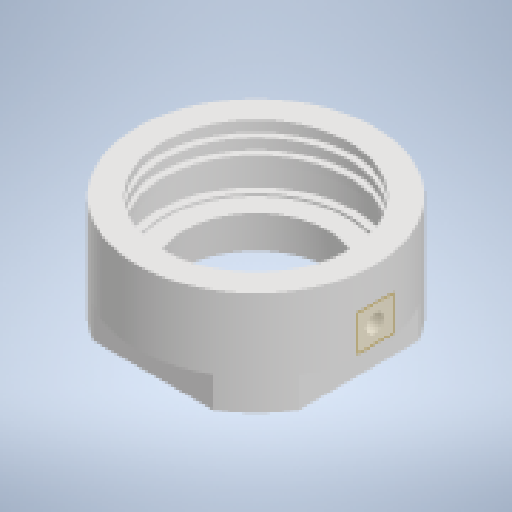
# Autodesk Inventor part: WashChamberConduit_1
Saved by Autodesk Inventor 2024 (Build 280153000, 153)
## iProperties
Created: 2025-02-06
Part Number: WashChamberConduit_1
Material: Generic
Document SubType Name: Modeling
Designer: Tommy Rohmann
Density: 1 g/cm^3
Appearance: Default
Author: Tommy Rohmann
Autodesk Inventor part; units mm, degrees
ref_plane "YZ Plane" through (0, 0, 0) normal (1, 0, 0) x (0, 1, 0)
ref_plane "XZ Plane" through (0, 0, 0) normal (0, 1, 0) x (-1, 0, 0)
ref_plane "XY Plane" through (0, 0, 0) normal (0, 0, 1) x (1, 0, 0)
sketch "WashChamberConduit" plane through (0, 0, 0) normal (0, 0, 1) x (1, 0, 0)
  line L0 (57.15, 1.0107) -> (61.9125, 1.0107)
  line L1 (57.15, -2.1643) -> (57.15, 31.7898)
  line L2 (57.785, 35.3007) -> (61.9125, 35.3007)
  line L3 (61.9125, 35.3007) -> (61.9125, 30.5382)
  line L4 (61.9125, 30.5382) -> (57.785, 30.5382)
  line L5 (57.785, 30.5382) -> (57.785, 25.7757)
  line L6 (57.785, 25.7757) -> (61.9125, 25.7757)
  line L7 (61.9125, 25.7757) -> (61.9125, 21.0132)
  line L8 (61.9125, 1.0107) -> (61.9125, 16.2507)
  line L9 (57.785, 35.3007) -> (57.785, 40.0632)
  line L10 (57.785, 40.0632) -> (73.9267, 40.0632)
  line L11 (73.9267, -5.3393) -> (63.7667, -5.3393)
  line L12 (63.7667, -5.3393) -> (63.7667, -24.3893)
  line L13 (61.9125, 21.0132) -> (57.785, 21.0132)
  line L14 (57.785, 21.0132) -> (57.785, 16.2507)
  line L15 (57.785, 16.2507) -> (61.9125, 16.2507)
  line L16 (0, 0) -> (0, 25.5104)
  line L17 (73.9267, -5.3393) -> (73.9267, 40.0632)
  line L18 (57.15, 1.0107) -> (57.15, -0.5768)
  line L19 (63.7667, -24.3893) -> (73.9267, -24.3893)
  line L20 (73.9267, -24.3893) -> (73.9267, -5.3393)
  line L21 (61.9125, 8.6307) -> (73.9267, 8.6307)
  line L22 (57.15, 1.0107) -> (63.8852, 1.0107)
  line L23 (57.15, -0.5768) -> (44.45, -0.5768)
  line L24 (44.45, -0.5768) -> (46.0375, -8.5143)
  line L25 (46.0375, -8.5143) -> (47.625, -16.4518)
  line L26 (47.625, -16.4518) -> (49.2125, -24.3893)
  line L27 (63.7667, -24.3893) -> (49.2125, -24.3893)
  point P0 (52.07, -10.4939)
  dimension "d9" = 0.635
  dimension "d12" = 4.7625
  dimension "d13" = 4.7625
  dimension "d17" = 15.24
  dimension "d41" = 10.16
  dimension "d42" = 12.0142
  dimension "d44" = 114.3
  dimension "WashConduitOD" = 147.8534
  dimension "d46" = 1.5875
  dimension "d65" = 19.05
  dimension "d232" = 92.075
  dimension "d233" = 95.25
  dimension "d234" = 23.8125
  dimension "ConduitHatchAngle" = 78.69
  dimension "ConduitHatchID" = 88.9
  measures "d9" distance between parallel lines of L1 L9
  measures "d12" distance between parallel lines of L1 L3
  measures "d13" distance between parallel lines of L2 L10
  measures "d17" distance between parallel lines of L15 L0
  measures "d41" distance between parallel lines of L17 L12
  measures "d42" distance between parallel lines of L17 L8
  measures "d44" diameter of L1 L16
  measures "WashConduitOD" diameter of L17 L16
  measures "d46" distance of L0.start L18.end
  measures "d65" distance between parallel lines of L19 L11
  measures "d232" diameter of L24.end L16
  measures "d233" diameter of L25.end L16
  measures "d234" distance from line of L23.end L27
  measures "ConduitHatchAngle" angle of L23 L24
  measures "ConduitHatchID" diameter of L23.end L16
derived "WashChamberLayout.ipt"
sketch "Sketch1" plane through (0, 0, 0) normal (0, 0, 1) x (1, 0, 0)
  line L0 (57.15, 1.0107) -> (61.9125, 1.0107)
  line L1 (57.15, -2.1643) -> (57.15, 31.7898)
  line L2 (57.785, 35.3007) -> (61.9125, 35.3007)
  line L3 (61.9125, 35.3007) -> (61.9125, 30.5382)
  line L4 (61.9125, 30.5382) -> (57.785, 30.5382)
  line L5 (57.785, 30.5382) -> (57.785, 25.7757)
  line L6 (57.785, 25.7757) -> (61.9125, 25.7757)
  line L7 (61.9125, 25.7757) -> (61.9125, 21.0132)
  line L8 (61.9125, 1.0107) -> (61.9125, 16.2507)
  line L9 (57.785, 35.3007) -> (57.785, 40.0632)
  line L10 (57.785, 40.0632) -> (73.9267, 40.0632)
  line L11 (73.9267, -5.3393) -> (63.7667, -5.3393)
  line L12 (63.7667, -5.3393) -> (63.7667, -24.3893)
  line L13 (61.9125, 21.0132) -> (57.785, 21.0132)
  line L14 (57.785, 21.0132) -> (57.785, 16.2507)
  line L15 (57.785, 16.2507) -> (61.9125, 16.2507)
  line L16 (0, 0) -> (0, 25.5104)
  line L17 (73.9267, -5.3393) -> (73.9267, 40.0632)
  line L18 (57.15, 1.0107) -> (57.15, -0.5768)
  line L19 (63.7667, -24.3893) -> (73.9267, -24.3893)
  line L20 (73.9267, -24.3893) -> (73.9267, -5.3393)
  line L21 (61.9125, 8.6307) -> (73.9267, 8.6307)
  line L22 (57.15, 1.0107) -> (63.8852, 1.0107)
  line L23 (57.15, -0.5768) -> (44.45, -0.5768)
  line L24 (44.45, -0.5768) -> (46.0375, -8.5143)
  line L25 (46.0375, -8.5143) -> (47.625, -16.4518)
  line L26 (47.625, -16.4518) -> (49.2125, -24.3893)
  line L27 (63.7667, -24.3893) -> (49.2125, -24.3893)
revolve "Revolution1" add sketch "Sketch1" angle 90 mid plane about axis through (0, 0, 0) along (0, 1, 0)
extrude "Extrusion1" cut sketch "Sketch1" along normal mid plane 249.2375 contours L20 L19 L12 L11
ref_plane "Work Plane1" through (73.9267, 8.6307, 0) normal (1, 0, 0) x (0, 1, 0)
pattern_circular "Circular Pattern1" count 4 over 360 about axis through (0, -10, 0) along (0, 1, 0)
sketch "Sketch2" plane through (73.9267, 8.6307, 0) normal (1, 0, 0) x (0, 1, 0)
  circle A0 centre (0, 0) radius 5.4356
  point P0 (-8.6307, 0)
  dimension "d10" = 10.8712
  constraints: 1 centre point
  measures "d10" diameter of A0
extrude "Extrusion2" cut sketch "Sketch2" along normal mid plane 76.2
body "Solid1"
